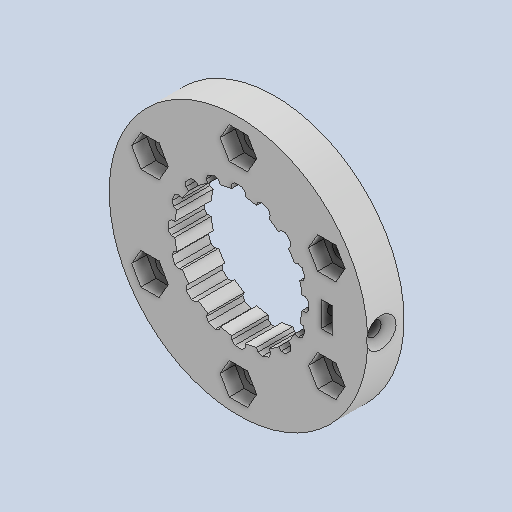
# Autodesk Inventor part: цил1
Saved by Autodesk Inventor 2024 (Build 280153000, 153)
## iProperties
Created: 2025-10-16
Part Number: цил1
Material: Типовые
Document SubType Name: Modeling
Designer: DELL
Density: 1 g/cm^3
Appearance: По умолчанию
Author: DELL
Autodesk Inventor part; units mm, degrees
ref_plane "YZ Plane" through (0, 0, 0) normal (1, 0, 0) x (0, 1, 0)
ref_plane "XZ Plane" through (0, 0, 0) normal (0, 1, 0) x (-1, 0, 0)
ref_plane "XY Plane" through (0, 0, 0) normal (0, 0, 1) x (1, 0, 0)
sketch "Эскиз1" plane through (0, 0, 0) normal (0, 0, 1) x (1, 0, 0)
  circle A0 centre (0, 0) radius 22.5 construction
  circle A1 centre (0, 0) radius 28.5
  circle A2 centre (0, 0) radius 14.1
  dimension "d1" = 45
  dimension "d7" = 6
  dimension "d10" = 28.2
  constraints: 3 centre point, 2 coincident
  measures "d1" diameter of A0
  measures "d7" radial gap between concentric circles of A0 A1
  measures "d10" diameter of A2
extrude "Выдавливание1" add sketch "Эскиз1" along normal blind 8
sketch "Эскиз2" plane through (0, 0, 8) normal (0, 0, 1) x (1, 0, 0)
  circle A0 centre (0, 0) radius 22.5 construction
  circle A1 centre (0, 22.5) radius 2.1
  dimension "d14" = 45
  dimension "d15" = 4.2
  constraints: 1 centre point, 1 coincident, 1 vertical alignment, 2 other
  measures "d15" diameter of A1
extrude "Выдавливание2" cut sketch "Эскиз2" against normal blind 10
sketch "Эскиз3" plane through (0, 0, 8) normal (0, 0, 1) x (1, 0, 0)
  circle A0 centre (0, 22.5) radius 2.1 projected
  line L0 (4.0415, 22.5) -> (2.0207, 19)
  line L1 (2.0207, 19) -> (-2.0207, 19)
  line L2 (-2.0207, 19) -> (-4.0415, 22.5)
  line L3 (-4.0415, 22.5) -> (-2.0207, 26)
  line L4 (-2.0207, 26) -> (2.0207, 26)
  line L5 (2.0207, 26) -> (4.0415, 22.5)
  point P0 (0, 0)
  point P1 (0, 19)
  dimension "d24" = 7
  constraints: 12 end point, 1 coincident, 1 midpoint, 13 other
  measures "d24" distance from line of point (0, 19) L4
extrude "Выдавливание3" cut sketch "Эскиз3" against normal blind 3.3
pattern_circular "Круговой массив1" count 6 over 360 about axis through (0, 0, 0) along (0, 0, 1) of "Выдавливание2", "Выдавливание3"
sketch "Эскиз4" plane through (0, 0, 8) normal (0, 0, 1) x (1, 0, 0)
  line L0 (0, 0) -> (43.2102, 0) construction
  line L1 (21.5063, 7.75) -> (17.4648, 7.75) construction
  line L2 (21.5063, 7.75) -> (17.4648, 7.75) projected
  line L3 (19.4856, 7.75) -> (19.4856, -6.0853) construction
  line L4 (20.7356, 2.8) -> (18.2356, 2.8)
  line L5 (18.2356, 2.8) -> (18.2356, -2.8)
  line L6 (18.2356, -2.8) -> (20.7356, -2.8)
  line L7 (20.7356, -2.8) -> (20.7356, 2.8)
  line L8 (20.7356, 2.8) -> (18.2356, -2.8) construction
  line L9 (18.2356, 2.8) -> (20.7356, -2.8) construction
  point P0 (19.4856, 0)
  dimension "d27" = 2.5
  dimension "d28" = 5.6
  constraints: 16 end point, 3 midpoint, 2 horizontal, 2 parallel, 2 point on line, 1 perpendicular, 1 vertical
  measures "d27" distance of L6.end L5.end
  measures "d28" distance of L5.end L4.end
extrude "Выдавливание4" cut sketch "Эскиз4" against normal blind 6
sketch "Эскиз5" plane through (18.2356, -2.8, 8) normal (1, 0, 0) x (0, 0, -1)
  line L0 (0, -4.95) -> (3.3, -4.95) construction
  circle A0 centre (3, 2.7761) radius 1.6
  line L1 (0, -11.3) -> (0, 16.9) projected
  dimension "d31" = 3.2
  dimension "d32" = 3
  constraints: 1 centre point
  measures "d31" diameter of A0
  measures "d32" distance from line of L1 A0.centre
extrude "Выдавливание5" cut sketch "Эскиз5" along normal mid plane 30
chamfer "Фаска3" distance 1.65 angle 45 3 edges at (28.5, -0.012, 3.4) (28.4537, -1.6239, 5.009) (28.4564, 1.576, 5.0063)
sketch "Эскиз6" plane through (0, 0, 8) normal (0, 0, 1) x (1, 0, 0)
  circle A0 centre (0, 0) radius 14.1 projected
  line L0 (-1.5295, 14.8168) -> (-1.5295, 14.0168)
  line L1 (-1.5295, 14.0168) -> (1.4705, 14.0168)
  line L2 (1.4705, 14.0168) -> (1.4705, 14.8168)
  line L3 (0.7705, 15.5168) -> (-0.8295, 15.5168)
  line L4 (-1.5295, 15.5168) -> (1.4705, 14.0168) construction
  line L5 (-1.5295, 14.0168) -> (1.4705, 15.5168) construction
  line L6 (-0.8295, 15.5168) -> (-1.5295, 14.8168)
  line L7 (0.7705, 15.5168) -> (1.4705, 14.8168)
  line L8 (-5.2261, 14.6305) -> (-6.7043, 14.0182)
  line L9 (-6.7043, 14.0182) -> (-7.0832, 13.1036)
  line L10 (-6.777, 12.3645) -> (-4.5794, 14.8984) construction
  line L11 (-5.2261, 14.6305) -> (-4.3115, 14.2517)
  line L12 (-7.3511, 13.7504) -> (-4.0054, 13.5126) construction
  line L13 (-7.0832, 13.1036) -> (-6.777, 12.3645)
  line L14 (-6.777, 12.3645) -> (-4.0054, 13.5126)
  line L15 (-4.0054, 13.5126) -> (-4.3115, 14.2517)
  line L16 (-10.4272, 11.5169) -> (-11.5586, 10.3855)
  line L17 (-11.5586, 10.3855) -> (-11.5586, 9.3956)
  line L18 (-10.9929, 8.8299) -> (-9.9322, 12.0119) construction
  line L19 (-10.4272, 11.5169) -> (-9.4372, 11.5169)
  line L20 (-12.0535, 9.8905) -> (-8.8715, 10.9512) construction
  line L21 (-11.5586, 9.3956) -> (-10.9929, 8.8299)
  line L22 (-10.9929, 8.8299) -> (-8.8715, 10.9512)
  line L23 (-8.8715, 10.9512) -> (-9.4372, 11.5169)
  line L24 (-14.0408, 6.6499) -> (-14.6531, 5.1717)
  line L25 (-14.6531, 5.1717) -> (-14.2742, 4.2571)
  line L26 (-13.5351, 3.951) -> (-13.7729, 7.2966) construction
  line L27 (-14.0408, 6.6499) -> (-13.1262, 7.0287)
  line L28 (-14.921, 4.525) -> (-12.3871, 6.7226) construction
  line L29 (-14.2742, 4.2571) -> (-13.5351, 3.951)
  line L30 (-13.5351, 3.951) -> (-12.3871, 6.7226)
  line L31 (-12.3871, 6.7226) -> (-13.1262, 7.0287)
  line L32 (-15.5168, 0.7705) -> (-15.5168, -0.8295)
  line L33 (-15.5168, -0.8295) -> (-14.8168, -1.5295)
  line L34 (-14.0168, -1.5295) -> (-15.5168, 1.4705) construction
  line L35 (-15.5168, 0.7705) -> (-14.8168, 1.4705)
  line L36 (-15.5168, -1.5295) -> (-14.0168, 1.4705) construction
  line L37 (-14.8168, -1.5295) -> (-14.0168, -1.5295)
  line L38 (-14.0168, -1.5295) -> (-14.0168, 1.4705)
  line L39 (-14.0168, 1.4705) -> (-14.8168, 1.4705)
  line L40 (-14.6305, -5.2261) -> (-14.0182, -6.7043)
  line L41 (-14.0182, -6.7043) -> (-13.1036, -7.0832)
  line L42 (-12.3645, -6.777) -> (-14.8984, -4.5794) construction
  line L43 (-14.6305, -5.2261) -> (-14.2517, -4.3115)
  line L44 (-13.7504, -7.3511) -> (-13.5126, -4.0054) construction
  line L45 (-13.1036, -7.0832) -> (-12.3645, -6.777)
  line L46 (-12.3645, -6.777) -> (-13.5126, -4.0054)
  line L47 (-13.5126, -4.0054) -> (-14.2517, -4.3115)
  line L48 (-11.5169, -10.4272) -> (-10.3855, -11.5586)
  line L49 (-10.3855, -11.5586) -> (-9.3956, -11.5586)
  line L50 (-8.8299, -10.9929) -> (-12.0119, -9.9322) construction
  line L51 (-11.5169, -10.4272) -> (-11.5169, -9.4372)
  line L52 (-9.8905, -12.0535) -> (-10.9512, -8.8715) construction
  line L53 (-9.3956, -11.5586) -> (-8.8299, -10.9929)
  line L54 (-8.8299, -10.9929) -> (-10.9512, -8.8715)
  line L55 (-10.9512, -8.8715) -> (-11.5169, -9.4372)
  line L56 (-6.6499, -14.0408) -> (-5.1717, -14.6531)
  line L57 (-5.1717, -14.6531) -> (-4.2571, -14.2742)
  line L58 (-3.951, -13.5351) -> (-7.2966, -13.7729) construction
  line L59 (-6.6499, -14.0408) -> (-7.0287, -13.1262)
  line L60 (-4.525, -14.921) -> (-6.7226, -12.3871) construction
  line L61 (-4.2571, -14.2742) -> (-3.951, -13.5351)
  line L62 (-3.951, -13.5351) -> (-6.7226, -12.3871)
  line L63 (-6.7226, -12.3871) -> (-7.0287, -13.1262)
  line L64 (-0.7705, -15.5168) -> (0.8295, -15.5168)
  line L65 (0.8295, -15.5168) -> (1.5295, -14.8168)
  line L66 (1.5295, -14.0168) -> (-1.4705, -15.5168) construction
  line L67 (-0.7705, -15.5168) -> (-1.4705, -14.8168)
  line L68 (1.5295, -15.5168) -> (-1.4705, -14.0168) construction
  line L69 (1.5295, -14.8168) -> (1.5295, -14.0168)
  line L70 (1.5295, -14.0168) -> (-1.4705, -14.0168)
  line L71 (-1.4705, -14.0168) -> (-1.4705, -14.8168)
  line L72 (5.2261, -14.6305) -> (6.7043, -14.0182)
  line L73 (6.7043, -14.0182) -> (7.0832, -13.1036)
  line L74 (6.777, -12.3645) -> (4.5794, -14.8984) construction
  line L75 (5.2261, -14.6305) -> (4.3115, -14.2517)
  line L76 (7.3511, -13.7504) -> (4.0054, -13.5126) construction
  line L77 (7.0832, -13.1036) -> (6.777, -12.3645)
  line L78 (6.777, -12.3645) -> (4.0054, -13.5126)
  line L79 (4.0054, -13.5126) -> (4.3115, -14.2517)
  line L80 (10.4272, -11.5169) -> (11.5586, -10.3855)
  line L81 (11.5586, -10.3855) -> (11.5586, -9.3956)
  line L82 (10.9929, -8.8299) -> (9.9322, -12.0119) construction
  line L83 (10.4272, -11.5169) -> (9.4372, -11.5169)
  line L84 (12.0535, -9.8905) -> (8.8715, -10.9512) construction
  line L85 (11.5586, -9.3956) -> (10.9929, -8.8299)
  line L86 (10.9929, -8.8299) -> (8.8715, -10.9512)
  line L87 (8.8715, -10.9512) -> (9.4372, -11.5169)
  line L88 (14.0408, -6.6499) -> (14.6531, -5.1717)
  line L89 (14.6531, -5.1717) -> (14.2742, -4.2571)
  line L90 (13.5351, -3.951) -> (13.7729, -7.2966) construction
  line L91 (14.0408, -6.6499) -> (13.1262, -7.0287)
  line L92 (14.921, -4.525) -> (12.3871, -6.7226) construction
  line L93 (14.2742, -4.2571) -> (13.5351, -3.951)
  line L94 (13.5351, -3.951) -> (12.3871, -6.7226)
  line L95 (12.3871, -6.7226) -> (13.1262, -7.0287)
  line L96 (15.5168, -0.7705) -> (15.5168, 0.8295)
  line L97 (15.5168, 0.8295) -> (14.8168, 1.5295)
  line L98 (14.0168, 1.5295) -> (15.5168, -1.4705) construction
  line L99 (15.5168, -0.7705) -> (14.8168, -1.4705)
  line L100 (15.5168, 1.5295) -> (14.0168, -1.4705) construction
  line L101 (14.8168, 1.5295) -> (14.0168, 1.5295)
  line L102 (14.0168, 1.5295) -> (14.0168, -1.4705)
  line L103 (14.0168, -1.4705) -> (14.8168, -1.4705)
  line L104 (14.6305, 5.2261) -> (14.0182, 6.7043)
  line L105 (14.0182, 6.7043) -> (13.1036, 7.0832)
  line L106 (12.3645, 6.777) -> (14.8984, 4.5794) construction
  line L107 (14.6305, 5.2261) -> (14.2517, 4.3115)
  line L108 (13.7504, 7.3511) -> (13.5126, 4.0054) construction
  line L109 (13.1036, 7.0832) -> (12.3645, 6.777)
  line L110 (12.3645, 6.777) -> (13.5126, 4.0054)
  line L111 (13.5126, 4.0054) -> (14.2517, 4.3115)
  line L112 (11.5169, 10.4272) -> (10.3855, 11.5586)
  line L113 (10.3855, 11.5586) -> (9.3956, 11.5586)
  line L114 (8.8299, 10.9929) -> (12.0119, 9.9322) construction
  line L115 (11.5169, 10.4272) -> (11.5169, 9.4372)
  line L116 (9.8905, 12.0535) -> (10.9512, 8.8715) construction
  line L117 (9.3956, 11.5586) -> (8.8299, 10.9929)
  line L118 (8.8299, 10.9929) -> (10.9512, 8.8715)
  line L119 (10.9512, 8.8715) -> (11.5169, 9.4372)
  line L120 (6.6499, 14.0408) -> (5.1717, 14.6531)
  line L121 (5.1717, 14.6531) -> (4.2571, 14.2742)
  line L122 (3.951, 13.5351) -> (7.2966, 13.7729) construction
  line L123 (6.6499, 14.0408) -> (7.0287, 13.1262)
  line L124 (4.525, 14.921) -> (6.7226, 12.3871) construction
  line L125 (4.2571, 14.2742) -> (3.951, 13.5351)
  line L126 (3.951, 13.5351) -> (6.7226, 12.3871)
  line L127 (6.7226, 12.3871) -> (7.0287, 13.1262)
  point P0 (-0.0295, 14.7668)
  dimension "d38" = 3
  dimension "d39" = 1.5
  dimension "d40" = 0.7
  dimension "d41" = 0.7
  dimension "d42" = 0.7
  dimension "d43" = 0.7
  dimension "d46" = 360
  constraints: 256 end point, 64 point on line, 2 midpoint, 2 parallel, 1 perpendicular, 1 vertical, 259 other
  measures "d38" distance of L1.end L0.end
  measures "d39" distance of L1.end L5.end
  measures "d40" distance of L3.end L4.start
  measures "d41" distance of L0.start L4.start
  measures "d42" distance of L3.start L5.end
  measures "d43" distance of L2.end L5.end
extrude "Выдавливание6" cut sketch "Эскиз6" against normal blind 10 contours A0 L103 L102 | A0 L101 L97 L96 L99 L103 | L111 L110 A0 | A0 L109 L105 L104 L107 L111 | L93 L89 L88 L91 L95 A0 | A0 L95 L94 | L119 L118 A0 | A0 L117 L113 L112 L115 L119 | L85 L81 L80 L83 L87 A0 | A0 L87 L86 | L127 L126 A0 | A0 L125 L121 L120 L123 L127 | L77 L73 L72 L75 L79 A0 | A0 L79 L78 | L2 L1 A0 | A0 L0 L6 L3 L7 L2 | L69 L65 L64 L67 L71 A0 | A0 L71 L70 | L15 L14 A0 | A0 L13 L9 L8 L11 L15 | L61 L57 L56 L59 L63 A0 | A0 L63 L62 | L23 L22 A0 | A0 L21 L17 L16 L19 L23 | L53 L49 L48 L51 L55 A0 | A0 L55 L54 | L31 L30 A0 | A0 L29 L25 L24 L27 L31 | L45 L41 L40 L43 L47 A0 | A0 L47 L46 | L39 L38 A0 | A0 L37 L33 L32 L35 L39
chamfer "Фаска4" distance 2.2 angle 45 6 edges at (-20.5356, 9.4313, 0) (-18.4356, -13.0687, 0) (2.1, -22.5, 0) (20.5356, -9.4313, 0) (18.4356, 13.0687, 0) (-2.1, 22.5, 0)
equation "\"d41\" = d40"
equation "\"d42\" = d40"
equation "\"d43\" = d42"
